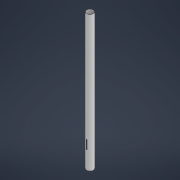
# Autodesk Inventor part: Shaft connecting chassis updated 1-19
Saved by Autodesk Inventor 2022 (Build 260153000, 153)
## iProperties
Created: 2022-01-19
Part Number: Shaft connecting chassis updated 1-19
Material: Generic
Document SubType Name: Modeling
Designer: raymo
Density: 1 g/cm^3
Appearance: Default
Author: raymo
Autodesk Inventor part; units mm, degrees
ref_plane "YZ Plane" through (0, 0, 0) normal (1, 0, 0) x (0, 1, 0)
ref_plane "XZ Plane" through (0, 0, 0) normal (0, 1, 0) x (-1, 0, 0)
sketch "Sketch1" plane through (0, 0, 0) normal (0, 1, 0) x (-1, 0, 0)
  circle A0 centre (0, 0) radius 19.05
  dimension "d0" = 38.1
  constraints: 1 centre point, 1 coincident
  measures "d0" diameter of A0
extrude "Extrusion1" add sketch "Sketch1" along normal blind 762
sketch "Sketch2" plane through (0, 762, 0) normal (0, 1, 0) x (1, 0, 0)
  circle A0 centre (0, 0) radius 18
  dimension "d3" = 36
  constraints: 1 centre point, 1 coincident
  measures "d3" diameter of A0
extrude "Extrusion2" cut sketch "Sketch2" along normal through all both and the other way through all
ref_plane "Work Plane1" through (0, 0, 29.95) normal (0, 0, 1) x (1, 0, 0)
sketch "Sketch3" plane through (0, 0, 29.95) normal (0, 0, 1) x (1, 0, 0)
  line L0 (0, 0) -> (0, 100)
  line L1 (-18, 100) -> (18, 100) projected
  line L2 (-2.3812, 100) -> (2.3812, 100)
  line L3 (2.3812, 100) -> (2.3813, 150)
  line L4 (2.3813, 150) -> (-2.3812, 150)
  line L5 (-2.3812, 150) -> (-2.3812, 100)
  dimension "d15" = 4.7625
  dimension "d16" = 50
  constraints: 10 end point, 2 midpoint, 2 parallel, 1 horizontal, 1 perpendicular, 1 point on line, 1 vertical
  measures "d15" distance of L3.end L4.end
  measures "d16" distance of L2.end L3.end
extrude "Extrusion3" cut sketch "Sketch3" against normal blind 29.95
sketch "Sketch4" plane through (0, 0, 0) normal (0, -1, 0) x (1, 0, 0)
  circle A0 centre (0, 0) radius 19
  circle A1 centre (0, 0) radius 29.95
  dimension "d11" = 38
  constraints: 2 centre point, 2 coincident
  measures "d11" diameter of A0
body "Solid1"
